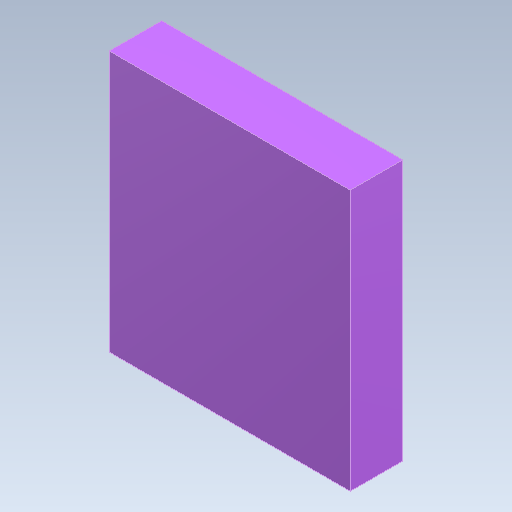
# Autodesk Inventor part: 78L12F
Saved by Autodesk Inventor 2021 (Build 250183000, 183)
## iProperties
Created: 2020-11-18
Part Number: 78L12F
Material: Generic
Document SubType Name: Modeling
Designer: Admin
Density: 1 g/cm^3
Appearance: SOT89, 78L12F
Author: Admin
Autodesk Inventor part; units mm, degrees
ref_plane "YZ Plane" through (0, 0, 0) normal (1, 0, 0) x (0, 1, 0)
ref_plane "XZ Plane" through (0, 0, 0) normal (0, 1, 0) x (-1, 0, 0)
ref_plane "XY Plane" through (0, 0, 0) normal (0, 0, 1) x (1, 0, 0)
sketch "SOT89, 78L12F_24" plane through (0, 0, 0) normal (0, 0, 1) x (1, 0, 0)
  line L0 (-2.2985, 2.2) -> (2.2985, 2.2)
  line L1 (2.2985, 2.2) -> (2.2985, -2.775)
  line L2 (2.2985, -2.775) -> (-2.2985, -2.775)
  line L3 (-2.2985, -2.775) -> (-2.2985, 2.2)
  constraints: 8 end point
extrude "Extrusion1" add sketch "SOT89, 78L12F_24" along normal blind 1
body "Solid1"
